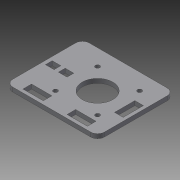
# Autodesk Inventor part: Air2D_Side_Motor
Saved by Autodesk Inventor 2014 (Build 180170000, 170)
## iProperties
Created: 2014-09-30
Part Number: Air2D_Side_Motor
Material: Generic
Document SubType Name: Modeling
Designer: ThatOtherGuy
Density: 1 g/cm^3
Appearance: Default
Author: ThatOtherGuy
Autodesk Inventor part; units mm, degrees
ref_plane "YZ Plane" through (0, 0, 0) normal (1, 0, 0) x (0, 1, 0)
ref_plane "XZ Plane" through (0, 0, 0) normal (0, 1, 0) x (-1, 0, 0)
ref_plane "XY Plane" through (0, 0, 0) normal (0, 0, 1) x (1, 0, 0)
sketch "Sketch1" plane through (0, 0, 0) normal (0, 0, 1) x (1, 0, 0)
  circle A0 centre (0, 0) radius 11.25
  circle A1 centre (-15.5, 15.5) radius 1.6
  circle A2 centre (15.5, 15.5) radius 1.6
  circle A3 centre (15.5, -15.5) radius 1.6
  circle A4 centre (-15.5, -15.5) radius 1.6
  line L0 (-19.231, 2.5) -> (-12.5, 2.5)
  line L1 (-12.5, 2.5) -> (-12.5, -2.5)
  line L2 (-12.5, -2.5) -> (-19.231, -2.5)
  line L3 (-19.231, -2.5) -> (-19.231, 2.5)
  line L4 (20, 7.5) -> (26.731, 7.5)
  line L5 (26.731, 7.5) -> (26.731, -7.5)
  line L6 (26.731, -7.5) -> (20, -7.5)
  line L7 (20, -7.5) -> (20, 7.5)
  line L8 (-30.769, 27.5) -> (29.231, 27.5)
  line L9 (29.231, 27.5) -> (29.231, -29.231)
  line L10 (29.231, -29.231) -> (-30.769, -29.231)
  line L11 (-30.769, -29.231) -> (-30.769, 27.5)
  line L12 (4.231, -20) -> (19.231, -20)
  line L13 (19.231, -20) -> (19.231, -26.731)
  line L14 (19.231, -26.731) -> (4.231, -26.731)
  line L15 (4.231, -26.731) -> (4.231, -20)
  line L16 (-29.162, 2.5) -> (-22.431, 2.5)
  line L17 (-22.431, 2.5) -> (-22.431, -2.5)
  line L18 (-22.431, -2.5) -> (-29.162, -2.5)
  line L19 (-29.162, -2.5) -> (-29.162, 2.5)
  line L20 (-20.769, -20) -> (-5.769, -20)
  line L21 (-5.769, -20) -> (-5.769, -26.731)
  line L22 (-5.769, -26.731) -> (-20.769, -26.731)
  line L23 (-20.769, -26.731) -> (-20.769, -20)
  point P0 (-12.5, 0)
  point P1 (20, 0)
  dimension "d0" = 22.5
  dimension "d1" = 3.2
  dimension "d2" = 31
  dimension "d3" = 31
  dimension "d4" = 15.5
  dimension "d5" = 15.5
  dimension "d6" = 32.5
  dimension "d7" = 20
  dimension "d8" = 5
  dimension "d9" = 6.731
  dimension "d13" = 20
  dimension "d17" = 2.5
  dimension "d18" = 20
  dimension "d19" = 2.5
  dimension "d20" = 3.2
  dimension "d25" = 15
  dimension "d26" = 10
  dimension "d28" = 60
  dimension "d29" = 10
  constraints: 48 end point, 12 parallel, 7 equal length, 6 horizontal, 6 perpendicular, 5 centre point, 4 horizontal alignment, 3 equal radius, 2 collinear, 2 midpoint, 2 vertical alignment, 1 coincident
  measures "d0" diameter of A0
  measures "d1" diameter of A1
  measures "d2" distance of A4.centre A1.centre
  measures "d3" distance of A1.centre A2.centre
  measures "d4" horizontal distance of point (0, 0) A1.centre
  measures "d5" horizontal distance of A1.centre point (0, 0)
  measures "d6" distance between parallel lines of L1 L7
  measures "d7" distance from line of L7 point (0, 0)
  measures "d8" distance of L2.end L0.start
  measures "d9" distance of L4.start L4.end
  measures "d13" distance from line of L12 point (0, 0)
  measures "d17" distance between parallel lines of L14 L10
  measures "d18" distance between parallel lines of L4 L8
  measures "d19" distance between parallel lines of L5 L9
  measures "d20" distance between parallel lines of L17 L3
  measures "d25" distance of L6.end L4.start
  measures "d26" distance between parallel lines of L9 L13
  measures "d28" distance of L8.start L8.end
  measures "d29" distance between parallel lines of L11 L23
extrude "Extrusion2" add sketch "Sketch1" along normal blind 6.731
fillet "Fillet2" radius 5 4 edges at (29.231, 27.5, 3.3655) (29.231, -29.231, 3.3655) (-30.769, -29.231, 3.3655) (-30.769, 27.5, 3.3655)
equation "\"d3\" = d2"
equation "\"d4\" = 0.5 * d2"
equation "\"d5\" = d4"
equation "\"d9\" = THICKB"
equation "\"d13\" = d7"
equation "\"d29\" = d26"
equation "\"d22\" = THICKB"
equation "\"THICKA\" = 3.175"
equation "\"THICKB\" = 6.731"
equation "\"THICKC\" = 12.7"
equation "\"BALLDIA\" = 12"
equation "\"MAGDIA\" = 9.5"
body "Solid2"
